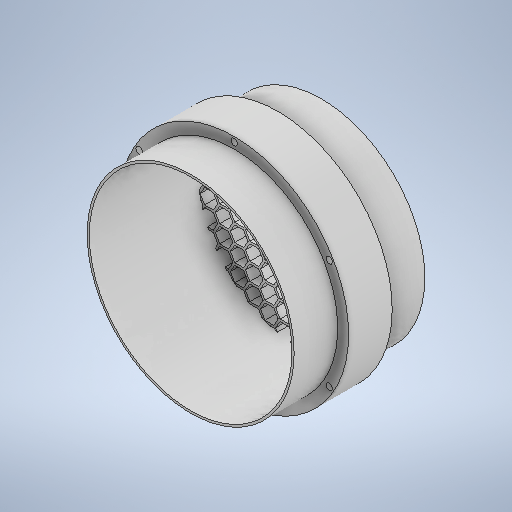
# Autodesk Inventor part: felga
Saved by Autodesk Inventor 2025.3 (Build 293356000, 356)
## iProperties
Created: 2026-03-06
Part Number: felga
Material: Generic
Document SubType Name: Modeling
Designer: ksawe
Density: 1 g/cm^3
Appearance: Default
Author: ksawe
Autodesk Inventor part; units mm, degrees
(part 1 of 2)
ref_plane "YZ Plane" through (0, 0, 0) normal (1, 0, 0) x (0, 1, 0)
ref_plane "XZ Plane" through (0, 0, 0) normal (0, 1, 0) x (-1, 0, 0)
sketch "Sketch8" plane through (0, 0, 0) normal (0, 0, 1) x (1, 0, 0)
  circle A0 centre (0, 0) radius 47.5
  dimension "d29" = 95
  constraints: 1 centre point, 1 coincident
  measures "d29" diameter of A0
extrude "Extrusion5" add sketch "Sketch8" along normal blind 60
ref_plane "Work Plane2" through (0, 0, 30) normal (0, 0, 1) x (1, 0, 0)
sketch "Sketch9" plane through (0, 0, 30) normal (0, 0, 1) x (1, 0, 0)
  circle A0 centre (0, 0) radius 52.5
  dimension "d33" = 105
  constraints: 1 centre point, 1 coincident
  measures "d33" diameter of A0
extrude "Extrusion6" add sketch "Sketch9" along normal mid plane 20
sketch "Sketch10" plane through (0, 0, 60) normal (0, 0, 1) x (1, 0, 0)
  circle A0 centre (0, 0) radius 46.5
  dimension "d36" = 93
  constraints: 1 centre point, 1 coincident
  measures "d36" diameter of A0
extrude "Extrusion7" cut sketch "Sketch10" against normal blind 50
sketch "Sketch14" plane through (0, 0, 0) normal (0, 0, -1) x (-1, 0, 0)
  line L0 (-2.0283, -3.4956) -> (-4.0414, 0.0088)
  line L1 (-4.0414, 0.0088) -> (-2.0131, 3.5044)
  line L2 (-2.0131, 3.5044) -> (2.0283, 3.4956)
  line L3 (2.0283, 3.4956) -> (4.0414, -0.0088)
  line L4 (4.0414, -0.0088) -> (2.0131, -3.5044)
  line L5 (2.0131, -3.5044) -> (-2.0283, -3.4956)
  line L6 (0, 0) -> (8.9984, 0) construction
  line L7 (0, 3.5) -> (0, 12.1066)
  line L8 (3.0311, -1.75) -> (7.7928, -4.4992)
  line L9 (4.0414, 7.9912) -> (2.0131, 4.4956)
  line L10 (2.0283, 11.4956) -> (4.0414, 7.9912)
  line L11 (-2.0131, 11.5044) -> (2.0283, 11.4956)
  line L12 (-4.0414, 8.0088) -> (-2.0131, 11.5044)
  line L13 (-2.0283, 4.5044) -> (-4.0414, 8.0088)
  line L14 (2.0131, 4.4956) -> (-2.0283, 4.5044)
  line L15 (4.0414, -8.0088) -> (2.0131, -11.5044)
  line L16 (2.0283, -4.5044) -> (4.0414, -8.0088)
  line L17 (-2.0131, -4.4956) -> (2.0283, -4.5044)
  line L18 (-4.0414, -7.9912) -> (-2.0131, -4.4956)
  line L19 (-2.0283, -11.4956) -> (-4.0414, -7.9912)
  line L20 (2.0131, -11.5044) -> (-2.0283, -11.4956)
  line L21 (4.0414, 15.9912) -> (2.0131, 12.4956)
  line L22 (2.0283, 19.4956) -> (4.0414, 15.9912)
  line L23 (-2.0131, 19.5044) -> (2.0283, 19.4956)
  line L24 (-4.0414, 16.0088) -> (-2.0131, 19.5044)
  line L25 (-2.0283, 12.5044) -> (-4.0414, 16.0088)
  line L26 (2.0131, 12.4956) -> (-2.0283, 12.5044)
  line L27 (4.0414, -16.0088) -> (2.0131, -19.5044)
  line L28 (2.0283, -12.5044) -> (4.0414, -16.0088)
  line L29 (-2.0131, -12.4956) -> (2.0283, -12.5044)
  line L30 (-4.0414, -15.9912) -> (-2.0131, -12.4956)
  line L31 (-2.0283, -19.4956) -> (-4.0414, -15.9912)
  line L32 (2.0131, -19.5044) -> (-2.0283, -19.4956)
  line L33 (4.0414, 23.9912) -> (2.0131, 20.4956)
  line L34 (2.0283, 27.4956) -> (4.0414, 23.9912)
  line L35 (-2.0131, 27.5044) -> (2.0283, 27.4956)
  line L36 (-4.0414, 24.0088) -> (-2.0131, 27.5044)
  line L37 (-2.0283, 20.5044) -> (-4.0414, 24.0088)
  line L38 (2.0131, 20.4956) -> (-2.0283, 20.5044)
  line L39 (4.0414, -24.0088) -> (2.0131, -27.5044)
  line L40 (2.0283, -20.5044) -> (4.0414, -24.0088)
  line L41 (-2.0131, -20.4956) -> (2.0283, -20.5044)
  line L42 (-4.0414, -23.9912) -> (-2.0131, -20.4956)
  line L43 (-2.0283, -27.4956) -> (-4.0414, -23.9912)
  line L44 (2.0131, -27.5044) -> (-2.0283, -27.4956)
  line L45 (4.0414, 31.9912) -> (2.0131, 28.4956)
  line L46 (2.0283, 35.4956) -> (4.0414, 31.9912)
  line L47 (-2.0131, 35.5044) -> (2.0283, 35.4956)
  line L48 (-4.0414, 32.0088) -> (-2.0131, 35.5044)
  line L49 (-2.0283, 28.5044) -> (-4.0414, 32.0088)
  line L50 (2.0131, 28.4956) -> (-2.0283, 28.5044)
  line L51 (4.0414, -32.0088) -> (2.0131, -35.5044)
  line L52 (2.0283, -28.5044) -> (4.0414, -32.0088)
  line L53 (-2.0131, -28.4956) -> (2.0283, -28.5044)
  line L54 (-4.0414, -31.9912) -> (-2.0131, -28.4956)
  line L55 (-2.0283, -35.4956) -> (-4.0414, -31.9912)
  line L56 (2.0131, -35.5044) -> (-2.0283, -35.4956)
  line L57 (4.0414, 39.9912) -> (2.0131, 36.4956)
  line L58 (2.0283, 43.4956) -> (4.0414, 39.9912)
  line L59 (-2.0131, 43.5044) -> (2.0283, 43.4956)
  line L60 (-4.0414, 40.0088) -> (-2.0131, 43.5044)
  line L61 (-2.0283, 36.5044) -> (-4.0414, 40.0088)
  line L62 (2.0131, 36.4956) -> (-2.0283, 36.5044)
  line L63 (4.0414, -40.0088) -> (2.0131, -43.5044)
  line L64 (2.0283, -36.5044) -> (4.0414, -40.0088)
  line L65 (-2.0131, -36.4956) -> (2.0283, -36.5044)
  line L66 (-4.0414, -39.9912) -> (-2.0131, -36.4956)
  line L67 (-2.0283, -43.4956) -> (-4.0414, -39.9912)
  line L68 (2.0131, -43.5044) -> (-2.0283, -43.4956)
  line L69 (4.0414, 47.9912) -> (2.0131, 44.4956)
  line L70 (2.0283, 51.4956) -> (4.0414, 47.9912)
  line L71 (-2.0131, 51.5044) -> (2.0283, 51.4956)
  line L72 (-4.0414, 48.0088) -> (-2.0131, 51.5044)
  line L73 (-2.0283, 44.5044) -> (-4.0414, 48.0088)
  line L74 (2.0131, 44.4956) -> (-2.0283, 44.5044)
  line L75 (4.0414, -48.0088) -> (2.0131, -51.5044)
  line L76 (2.0283, -44.5044) -> (4.0414, -48.0088)
  line L77 (-2.0131, -44.4956) -> (2.0283, -44.5044)
  line L78 (-4.0414, -47.9912) -> (-2.0131, -44.4956)
  line L79 (-2.0283, -51.4956) -> (-4.0414, -47.9912)
  line L80 (2.0131, -51.5044) -> (-2.0283, -51.4956)
  line L81 (4.0414, 55.9912) -> (2.0131, 52.4956)
  line L82 (2.0283, 59.4956) -> (4.0414, 55.9912)
  line L83 (-2.0131, 59.5044) -> (2.0283, 59.4956)
  line L84 (-4.0414, 56.0088) -> (-2.0131, 59.5044)
  line L85 (-2.0283, 52.5044) -> (-4.0414, 56.0088)
  line L86 (2.0131, 52.4956) -> (-2.0283, 52.5044)
  line L87 (4.0414, -56.0088) -> (2.0131, -59.5044)
  line L88 (2.0283, -52.5044) -> (4.0414, -56.0088)
  line L89 (-2.0131, -52.4956) -> (2.0283, -52.5044)
  line L90 (-4.0414, -55.9912) -> (-2.0131, -52.4956)
  line L91 (-2.0283, -59.4956) -> (-4.0414, -55.9912)
  line L92 (2.0131, -59.5044) -> (-2.0283, -59.4956)
  line L93 (10.9696, -4.0088) -> (8.9413, -7.5044)
  line L94 (8.9565, -0.5044) -> (10.9696, -4.0088)
  line L95 (4.9151, -0.4956) -> (8.9565, -0.5044)
  line L96 (2.8868, -3.9912) -> (4.9151, -0.4956)
  line L97 (4.8999, -7.4956) -> (2.8868, -3.9912)
  line L98 (8.9413, -7.5044) -> (4.8999, -7.4956)
  line L99 (10.9696, 3.9912) -> (8.9413, 0.4956)
  line L100 (8.9565, 7.4956) -> (10.9696, 3.9912)
  line L101 (4.9151, 7.5044) -> (8.9565, 7.4956)
  line L102 (2.8868, 4.0088) -> (4.9151, 7.5044)
  line L103 (4.8999, 0.5044) -> (2.8868, 4.0088)
  line L104 (8.9413, 0.4956) -> (4.8999, 0.5044)
  line L105 (10.9696, -12.0088) -> (8.9413, -15.5044)
  line L106 (8.9565, -8.5044) -> (10.9696, -12.0088)
  line L107 (4.9151, -8.4956) -> (8.9565, -8.5044)
  line L108 (2.8868, -11.9912) -> (4.9151, -8.4956)
  line L109 (4.8999, -15.4956) -> (2.8868, -11.9912)
  line L110 (8.9413, -15.5044) -> (4.8999, -15.4956)
  line L111 (10.9696, 11.9912) -> (8.9413, 8.4956)
  line L112 (8.9565, 15.4956) -> (10.9696, 11.9912)
  line L113 (4.9151, 15.5044) -> (8.9565, 15.4956)
  line L114 (2.8868, 12.0088) -> (4.9151, 15.5044)
  line L115 (4.8999, 8.5044) -> (2.8868, 12.0088)
  line L116 (8.9413, 8.4956) -> (4.8999, 8.5044)
  line L117 (10.9696, -20.0088) -> (8.9413, -23.5044)
  line L118 (8.9565, -16.5044) -> (10.9696, -20.0088)
  line L119 (4.9151, -16.4956) -> (8.9565, -16.5044)
  line L120 (2.8868, -19.9912) -> (4.9151, -16.4956)
  line L121 (4.8999, -23.4956) -> (2.8868, -19.9912)
  line L122 (8.9413, -23.5044) -> (4.8999, -23.4956)
  line L123 (10.9696, 19.9912) -> (8.9413, 16.4956)
  line L124 (8.9565, 23.4956) -> (10.9696, 19.9912)
  line L125 (4.9151, 23.5044) -> (8.9565, 23.4956)
  line L126 (2.8868, 20.0088) -> (4.9151, 23.5044)
  line L127 (4.8999, 16.5044) -> (2.8868, 20.0088)
  line L128 (8.9413, 16.4956) -> (4.8999, 16.5044)
  line L129 (10.9696, -28.0088) -> (8.9413, -31.5044)
  line L130 (8.9565, -24.5044) -> (10.9696, -28.0088)
  line L131 (4.9151, -24.4956) -> (8.9565, -24.5044)
  line L132 (2.8868, -27.9912) -> (4.9151, -24.4956)
  line L133 (4.8999, -31.4956) -> (2.8868, -27.9912)
  line L134 (8.9413, -31.5044) -> (4.8999, -31.4956)
  line L135 (10.9696, 27.9912) -> (8.9413, 24.4956)
  line L136 (8.9565, 31.4956) -> (10.9696, 27.9912)
  line L137 (4.9151, 31.5044) -> (8.9565, 31.4956)
  line L138 (2.8868, 28.0088) -> (4.9151, 31.5044)
  line L139 (4.8999, 24.5044) -> (2.8868, 28.0088)
  line L140 (8.9413, 24.4956) -> (4.8999, 24.5044)
  line L141 (10.9696, -36.0088) -> (8.9413, -39.5044)
  line L142 (8.9565, -32.5044) -> (10.9696, -36.0088)
  line L143 (4.9151, -32.4956) -> (8.9565, -32.5044)
  line L144 (2.8868, -35.9912) -> (4.9151, -32.4956)
  line L145 (4.8999, -39.4956) -> (2.8868, -35.9912)
  line L146 (8.9413, -39.5044) -> (4.8999, -39.4956)
  line L147 (10.9696, 35.9912) -> (8.9413, 32.4956)
  line L148 (8.9565, 39.4956) -> (10.9696, 35.9912)
  line L149 (4.9151, 39.5044) -> (8.9565, 39.4956)
  line L150 (2.8868, 36.0088) -> (4.9151, 39.5044)
  line L151 (4.8999, 32.5044) -> (2.8868, 36.0088)
  line L152 (8.9413, 32.4956) -> (4.8999, 32.5044)
  line L153 (10.9696, -44.0088) -> (8.9413, -47.5044)
  line L154 (8.9565, -40.5044) -> (10.9696, -44.0088)
  line L155 (4.9151, -40.4956) -> (8.9565, -40.5044)
  line L156 (2.8868, -43.9912) -> (4.9151, -40.4956)
  line L157 (4.8999, -47.4956) -> (2.8868, -43.9912)
  line L158 (8.9413, -47.5044) -> (4.8999, -47.4956)
  line L159 (10.9696, 43.9912) -> (8.9413, 40.4956)
  line L160 (8.9565, 47.4956) -> (10.9696, 43.9912)
  line L161 (4.9151, 47.5044) -> (8.9565, 47.4956)
  line L162 (2.8868, 44.0088) -> (4.9151, 47.5044)
  line L163 (4.8999, 40.5044) -> (2.8868, 44.0088)
  line L164 (8.9413, 40.4956) -> (4.8999, 40.5044)
  line L165 (10.9696, -52.0088) -> (8.9413, -55.5044)
  line L166 (8.9565, -48.5044) -> (10.9696, -52.0088)
  line L167 (4.9151, -48.4956) -> (8.9565, -48.5044)
  line L168 (2.8868, -51.9912) -> (4.9151, -48.4956)
  line L169 (4.8999, -55.4956) -> (2.8868, -51.9912) construction
  line L170 (8.9413, -55.5044) -> (4.8999, -55.4956)
  line L171 (10.9696, 51.9912) -> (8.9413, 48.4956)
  line L172 (8.9565, 55.4956) -> (10.9696, 51.9912)
  line L173 (4.9151, 55.5044) -> (8.9565, 55.4956)
  line L174 (2.8868, 52.0088) -> (4.9151, 55.5044)
  line L175 (4.8999, 48.5044) -> (2.8868, 52.0088)
  line L176 (8.9413, 48.4956) -> (4.8999, 48.5044)
  line L177 (10.9696, -60.0088) -> (8.9413, -63.5044)
  line L178 (8.9565, -56.5044) -> (10.9696, -60.0088)
  line L179 (4.9151, -56.4956) -> (8.9565, -56.5044)
  line L180 (2.8868, -59.9912) -> (4.9151, -56.4956)
  line L181 (4.8999, -63.4956) -> (2.8868, -59.9912)
  line L182 (8.9413, -63.5044) -> (4.8999, -63.4956)
  line L183 (-2.8868, 3.9912) -> (-4.9151, 0.4956)
  line L184 (-4.8999, 7.4956) -> (-2.8868, 3.9912)
  line L185 (-8.9413, 7.5044) -> (-4.8999, 7.4956)
  line L186 (-10.9696, 4.0088) -> (-8.9413, 7.5044)
  line L187 (-8.9565, 0.5044) -> (-10.9696, 4.0088)
  line L188 (-4.9151, 0.4956) -> (-8.9565, 0.5044)
  line L189 (-2.8868, 11.9912) -> (-4.9151, 8.4956)
  line L190 (-4.8999, 15.4956) -> (-2.8868, 11.9912)
  line L191 (-8.9413, 15.5044) -> (-4.8999, 15.4956)
  line L192 (-10.9696, 12.0088) -> (-8.9413, 15.5044)
  line L193 (-8.9565, 8.5044) -> (-10.9696, 12.0088)
  line L194 (-4.9151, 8.4956) -> (-8.9565, 8.5044)
  line L195 (-2.8868, -4.0088) -> (-4.9151, -7.5044)
  line L196 (-4.8999, -0.5044) -> (-2.8868, -4.0088)
  line L197 (-8.9413, -0.4956) -> (-4.8999, -0.5044)
  line L198 (-10.9696, -3.9912) -> (-8.9413, -0.4956)
  line L199 (-8.9565, -7.4956) -> (-10.9696, -3.9912)
  line L200 (-4.9151, -7.5044) -> (-8.9565, -7.4956)
  line L201 (-2.8868, 19.9912) -> (-4.9151, 16.4956)
  line L202 (-4.8999, 23.4956) -> (-2.8868, 19.9912)
  line L203 (-8.9413, 23.5044) -> (-4.8999, 23.4956)
  line L204 (-10.9696, 20.0088) -> (-8.9413, 23.5044)
  line L205 (-8.9565, 16.5044) -> (-10.9696, 20.0088)
  line L206 (-4.9151, 16.4956) -> (-8.9565, 16.5044)
  line L207 (-2.8868, -12.0088) -> (-4.9151, -15.5044)
  line L208 (-4.8999, -8.5044) -> (-2.8868, -12.0088)
  line L209 (-8.9413, -8.4956) -> (-4.8999, -8.5044)
  line L210 (-10.9696, -11.9912) -> (-8.9413, -8.4956)
  line L211 (-8.9565, -15.4956) -> (-10.9696, -11.9912)
  line L212 (-4.9151, -15.5044) -> (-8.9565, -15.4956)
  line L213 (-2.8868, 27.9912) -> (-4.9151, 24.4956)
  line L214 (-4.8999, 31.4956) -> (-2.8868, 27.9912)
  line L215 (-8.9413, 31.5044) -> (-4.8999, 31.4956)
  line L216 (-10.9696, 28.0088) -> (-8.9413, 31.5044)
  line L217 (-8.9565, 24.5044) -> (-10.9696, 28.0088)
  line L218 (-4.9151, 24.4956) -> (-8.9565, 24.5044)
  line L219 (-2.8868, -20.0088) -> (-4.9151, -23.5044)
  line L220 (-4.8999, -16.5044) -> (-2.8868, -20.0088)
  line L221 (-8.9413, -16.4956) -> (-4.8999, -16.5044)
  line L222 (-10.9696, -19.9912) -> (-8.9413, -16.4956)
  line L223 (-8.9565, -23.4956) -> (-10.9696, -19.9912)
  line L224 (-4.9151, -23.5044) -> (-8.9565, -23.4956)
  line L225 (-2.8868, 35.9912) -> (-4.9151, 32.4956)
  line L226 (-4.8999, 39.4956) -> (-2.8868, 35.9912)
  line L227 (-8.9413, 39.5044) -> (-4.8999, 39.4956)
  line L228 (-10.9696, 36.0088) -> (-8.9413, 39.5044)
  line L229 (-8.9565, 32.5044) -> (-10.9696, 36.0088)
  line L230 (-4.9151, 32.4956) -> (-8.9565, 32.5044)
  line L231 (-2.8868, -28.0088) -> (-4.9151, -31.5044)
  line L232 (-4.8999, -24.5044) -> (-2.8868, -28.0088)
  line L233 (-8.9413, -24.4956) -> (-4.8999, -24.5044)
  line L234 (-10.9696, -27.9912) -> (-8.9413, -24.4956)
  line L235 (-8.9565, -31.4956) -> (-10.9696, -27.9912)
  line L236 (-4.9151, -31.5044) -> (-8.9565, -31.4956)
  line L237 (-2.8868, 43.9912) -> (-4.9151, 40.4956)
  line L238 (-4.8999, 47.4956) -> (-2.8868, 43.9912)
  line L239 (-8.9413, 47.5044) -> (-4.8999, 47.4956)
  line L240 (-10.9696, 44.0088) -> (-8.9413, 47.5044)
  line L241 (-8.9565, 40.5044) -> (-10.9696, 44.0088)
  line L242 (-4.9151, 40.4956) -> (-8.9565, 40.5044)
  line L243 (-2.8868, -36.0088) -> (-4.9151, -39.5044)
  line L244 (-4.8999, -32.5044) -> (-2.8868, -36.0088)
  line L245 (-8.9413, -32.4956) -> (-4.8999, -32.5044)
  line L246 (-10.9696, -35.9912) -> (-8.9413, -32.4956)
  line L247 (-8.9565, -39.4956) -> (-10.9696, -35.9912)
  line L248 (-4.9151, -39.5044) -> (-8.9565, -39.4956)
  line L249 (-2.8868, 51.9912) -> (-4.9151, 48.4956)
  line L250 (-4.8999, 55.4956) -> (-2.8868, 51.9912)
  line L251 (-8.9413, 55.5044) -> (-4.8999, 55.4956)
  line L252 (-10.9696, 52.0088) -> (-8.9413, 55.5044)
  line L253 (-8.9565, 48.5044) -> (-10.9696, 52.0088)
  line L254 (-4.9151, 48.4956) -> (-8.9565, 48.5044)
  line L255 (-2.8868, -44.0088) -> (-4.9151, -47.5044)
  line L256 (-4.8999, -40.5044) -> (-2.8868, -44.0088)
  line L257 (-8.9413, -40.4956) -> (-4.8999, -40.5044)
  line L258 (-10.9696, -43.9912) -> (-8.9413, -40.4956)
  line L259 (-8.9565, -47.4956) -> (-10.9696, -43.9912)
  line L260 (-4.9151, -47.5044) -> (-8.9565, -47.4956)
  line L261 (-2.8868, 59.9912) -> (-4.9151, 56.4956)
  line L262 (-4.8999, 63.4956) -> (-2.8868, 59.9912)
  line L263 (-8.9413, 63.5044) -> (-4.8999, 63.4956)
  line L264 (-10.9696, 60.0088) -> (-8.9413, 63.5044)
  line L265 (-8.9565, 56.5044) -> (-10.9696, 60.0088)
  line L266 (-4.9151, 56.4956) -> (-8.9565, 56.5044)
  line L267 (-2.8868, -52.0088) -> (-4.9151, -55.5044)
  line L268 (-4.8999, -48.5044) -> (-2.8868, -52.0088)
  line L269 (-8.9413, -48.4956) -> (-4.8999, -48.5044)
  line L270 (-10.9696, -51.9912) -> (-8.9413, -48.4956)
  line L271 (-8.9565, -55.4956) -> (-10.9696, -51.9912)
  line L272 (-4.9151, -55.5044) -> (-8.9565, -55.4956)
  line L273 (17.8978, -8.0088) -> (15.8695, -11.5044)
  line L274 (15.8847, -4.5044) -> (17.8978, -8.0088)
  line L275 (11.8433, -4.4956) -> (15.8847, -4.5044)
  line L276 (9.815, -7.9912) -> (11.8433, -4.4956)
  line L277 (11.8281, -11.4956) -> (9.815, -7.9912)
  line L278 (15.8695, -11.5044) -> (11.8281, -11.4956)
  line L279 (17.8978, -0.0088) -> (15.8695, -3.5044)
  line L280 (15.8847, 3.4956) -> (17.8978, -0.0088)
  line L281 (11.8433, 3.5044) -> (15.8847, 3.4956)
  line L282 (9.815, 0.0088) -> (11.8433, 3.5044)
  line L283 (11.8281, -3.4956) -> (9.815, 0.0088)
  line L284 (15.8695, -3.5044) -> (11.8281, -3.4956)
  line L285 (17.8978, -16.0088) -> (15.8695, -19.5044)
  line L286 (15.8847, -12.5044) -> (17.8978, -16.0088)
  line L287 (11.8433, -12.4956) -> (15.8847, -12.5044)
  line L288 (9.815, -15.9912) -> (11.8433, -12.4956)
  line L289 (11.8281, -19.4956) -> (9.815, -15.9912)
  line L290 (15.8695, -19.5044) -> (11.8281, -19.4956)
  line L291 (17.8978, 7.9912) -> (15.8695, 4.4956)
  line L292 (15.8847, 11.4956) -> (17.8978, 7.9912)
  line L293 (11.8433, 11.5044) -> (15.8847, 11.4956)
  line L294 (9.815, 8.0088) -> (11.8433, 11.5044)
  line L295 (11.8281, 4.5044) -> (9.815, 8.0088)
  line L296 (15.8695, 4.4956) -> (11.8281, 4.5044)
  line L297 (17.8978, -24.0088) -> (15.8695, -27.5044)
  line L298 (15.8847, -20.5044) -> (17.8978, -24.0088)
  line L299 (11.8433, -20.4956) -> (15.8847, -20.5044)
  line L300 (9.815, -23.9912) -> (11.8433, -20.4956)
  line L301 (11.8281, -27.4956) -> (9.815, -23.9912)
  line L302 (15.8695, -27.5044) -> (11.8281, -27.4956)
  line L303 (17.8978, 15.9912) -> (15.8695, 12.4956)
  line L304 (15.8847, 19.4956) -> (17.8978, 15.9912)
  line L305 (11.8433, 19.5044) -> (15.8847, 19.4956)
  line L306 (9.815, 16.0088) -> (11.8433, 19.5044)
  line L307 (11.8281, 12.5044) -> (9.815, 16.0088)
  line L308 (15.8695, 12.4956) -> (11.8281, 12.5044)
  line L309 (17.8978, -32.0088) -> (15.8695, -35.5044)
  line L310 (15.8847, -28.5044) -> (17.8978, -32.0088)
  line L311 (11.8433, -28.4956) -> (15.8847, -28.5044)
  line L312 (9.815, -31.9912) -> (11.8433, -28.4956)
  line L313 (11.8281, -35.4956) -> (9.815, -31.9912)
  line L314 (15.8695, -35.5044) -> (11.8281, -35.4956)
  line L315 (17.8978, 23.9912) -> (15.8695, 20.4956)
  line L316 (15.8847, 27.4956) -> (17.8978, 23.9912)
  line L317 (11.8433, 27.5044) -> (15.8847, 27.4956)
  line L318 (9.815, 24.0088) -> (11.8433, 27.5044)
  line L319 (11.8281, 20.5044) -> (9.815, 24.0088)
  line L320 (15.8695, 20.4956) -> (11.8281, 20.5044)
  line L321 (17.8978, -40.0088) -> (15.8695, -43.5044)
  line L322 (15.8847, -36.5044) -> (17.8978, -40.0088)
  line L323 (11.8433, -36.4956) -> (15.8847, -36.5044)
  line L324 (9.815, -39.9912) -> (11.8433, -36.4956)
  line L325 (11.8281, -43.4956) -> (9.815, -39.9912)
  line L326 (15.8695, -43.5044) -> (11.8281, -43.4956)
  line L327 (17.8978, 31.9912) -> (15.8695, 28.4956)
  line L328 (15.8847, 35.4956) -> (17.8978, 31.9912)
  line L329 (11.8433, 35.5044) -> (15.8847, 35.4956)
  line L330 (9.815, 32.0088) -> (11.8433, 35.5044)
  line L331 (11.8281, 28.5044) -> (9.815, 32.0088)
  line L332 (15.8695, 28.4956) -> (11.8281, 28.5044)
  line L333 (17.8978, -48.0088) -> (15.8695, -51.5044)
  line L334 (15.8847, -44.5044) -> (17.8978, -48.0088)
  line L335 (11.8433, -44.4956) -> (15.8847, -44.5044)
  line L336 (9.815, -47.9912) -> (11.8433, -44.4956)
  line L337 (11.8281, -51.4956) -> (9.815, -47.9912)
  line L338 (15.8695, -51.5044) -> (11.8281, -51.4956)
  line L339 (17.8978, 39.9912) -> (15.8695, 36.4956)
  line L340 (15.8847, 43.4956) -> (17.8978, 39.9912)
  line L341 (11.8433, 43.5044) -> (15.8847, 43.4956)
  line L342 (9.815, 40.0088) -> (11.8433, 43.5044)
  line L343 (11.8281, 36.5044) -> (9.815, 40.0088)
  line L344 (15.8695, 36.4956) -> (11.8281, 36.5044)
  line L345 (17.8978, -56.0088) -> (15.8695, -59.5044)
  line L346 (15.8847, -52.5044) -> (17.8978, -56.0088)
  line L347 (11.8433, -52.4956) -> (15.8847, -52.5044)
  line L348 (9.815, -55.9912) -> (11.8433, -52.4956)
  line L349 (11.8281, -59.4956) -> (9.815, -55.9912)
  line L350 (15.8695, -59.5044) -> (11.8281, -59.4956)
  line L351 (17.8978, 47.9912) -> (15.8695, 44.4956)
  line L352 (15.8847, 51.4956) -> (17.8978, 47.9912)
  line L353 (11.8433, 51.5044) -> (15.8847, 51.4956)
  line L354 (9.815, 48.0088) -> (11.8433, 51.5044)
  line L355 (11.8281, 44.5044) -> (9.815, 48.0088)
  line L356 (15.8695, 44.4956) -> (11.8281, 44.5044)
  line L357 (17.8978, -64.0088) -> (15.8695, -67.5044)
  line L358 (15.8847, -60.5044) -> (17.8978, -64.0088)
  line L359 (11.8433, -60.4956) -> (15.8847, -60.5044)
  line L360 (9.815, -63.9912) -> (11.8433, -60.4956)
  line L361 (11.8281, -67.4956) -> (9.815, -63.9912)
  line L362 (15.8695, -67.5044) -> (11.8281, -67.4956)
  line L363 (-9.815, 7.9912) -> (-11.8433, 4.4956)
  line L364 (-11.8281, 11.4956) -> (-9.815, 7.9912)
  line L365 (-15.8695, 11.5044) -> (-11.8281, 11.4956)
  line L366 (-17.8978, 8.0088) -> (-15.8695, 11.5044)
  line L367 (-15.8847, 4.5044) -> (-17.8978, 8.0088)
  line L368 (-11.8433, 4.4956) -> (-15.8847, 4.5044)
  line L369 (-9.815, 15.9912) -> (-11.8433, 12.4956)
  line L370 (-11.8281, 19.4956) -> (-9.815, 15.9912)
  line L371 (-15.8695, 19.5044) -> (-11.8281, 19.4956)
  line L372 (-17.8978, 16.0088) -> (-15.8695, 19.5044)
  line L373 (-15.8847, 12.5044) -> (-17.8978, 16.0088)
  line L374 (-11.8433, 12.4956) -> (-15.8847, 12.5044)
  line L375 (-9.815, -0.0088) -> (-11.8433, -3.5044)
  line L376 (-11.8281, 3.4956) -> (-9.815, -0.0088)
  line L377 (-15.8695, 3.5044) -> (-11.8281, 3.4956)
  line L378 (-17.8978, 0.0088) -> (-15.8695, 3.5044)
  line L379 (-15.8847, -3.4956) -> (-17.8978, 0.0088)
  line L380 (-11.8433, -3.5044) -> (-15.8847, -3.4956)
  line L381 (-9.815, 23.9912) -> (-11.8433, 20.4956)
  line L382 (-11.8281, 27.4956) -> (-9.815, 23.9912)
  line L383 (-15.8695, 27.5044) -> (-11.8281, 27.4956)
  line L384 (-17.8978, 24.0088) -> (-15.8695, 27.5044)
  line L385 (-15.8847, 20.5044) -> (-17.8978, 24.0088)
  line L386 (-11.8433, 20.4956) -> (-15.8847, 20.5044)
  line L387 (-9.815, -8.0088) -> (-11.8433, -11.5044)
  line L388 (-11.8281, -4.5044) -> (-9.815, -8.0088)
  line L389 (-15.8695, -4.4956) -> (-11.8281, -4.5044)
  line L390 (-17.8978, -7.9912) -> (-15.8695, -4.4956)
  line L391 (-15.8847, -11.4956) -> (-17.8978, -7.9912)
  line L392 (-11.8433, -11.5044) -> (-15.8847, -11.4956)
  line L393 (-9.815, 31.9912) -> (-11.8433, 28.4956)
  line L394 (-11.8281, 35.4956) -> (-9.815, 31.9912)
  line L395 (-15.8695, 35.5044) -> (-11.8281, 35.4956)
  line L396 (-17.8978, 32.0088) -> (-15.8695, 35.5044)
  line L397 (-15.8847, 28.5044) -> (-17.8978, 32.0088)
  line L398 (-11.8433, 28.4956) -> (-15.8847, 28.5044)
  line L399 (-9.815, -16.0088) -> (-11.8433, -19.5044)
  line L400 (-11.8281, -12.5044) -> (-9.815, -16.0088)
  line L401 (-15.8695, -12.4956) -> (-11.8281, -12.5044)
  line L402 (-17.8978, -15.9912) -> (-15.8695, -12.4956)
  line L403 (-15.8847, -19.4956) -> (-17.8978, -15.9912)
  line L404 (-11.8433, -19.5044) -> (-15.8847, -19.4956)
  line L405 (-9.815, 39.9912) -> (-11.8433, 36.4956)
  line L406 (-11.8281, 43.4956) -> (-9.815, 39.9912)
  line L407 (-15.8695, 43.5044) -> (-11.8281, 43.4956)
  line L408 (-17.8978, 40.0088) -> (-15.8695, 43.5044)
  line L409 (-15.8847, 36.5044) -> (-17.8978, 40.0088)
  line L410 (-11.8433, 36.4956) -> (-15.8847, 36.5044)
  line L411 (-9.815, -24.0088) -> (-11.8433, -27.5044)
  line L412 (-11.8281, -20.5044) -> (-9.815, -24.0088)
  line L413 (-15.8695, -20.4956) -> (-11.8281, -20.5044)
  line L414 (-17.8978, -23.9912) -> (-15.8695, -20.4956)
  line L415 (-15.8847, -27.4956) -> (-17.8978, -23.9912)
  line L416 (-11.8433, -27.5044) -> (-15.8847, -27.4956)
  line L417 (-9.815, 47.9912) -> (-11.8433, 44.4956)
  line L418 (-11.8281, 51.4956) -> (-9.815, 47.9912)
  line L419 (-15.8695, 51.5044) -> (-11.8281, 51.4956)
  line L420 (-17.8978, 48.0088) -> (-15.8695, 51.5044)
  line L421 (-15.8847, 44.5044) -> (-17.8978, 48.0088)
  line L422 (-11.8433, 44.4956) -> (-15.8847, 44.5044)
  line L423 (-9.815, -32.0088) -> (-11.8433, -35.5044)
  line L424 (-11.8281, -28.5044) -> (-9.815, -32.0088)
  line L425 (-15.8695, -28.4956) -> (-11.8281, -28.5044)
  line L426 (-17.8978, -31.9912) -> (-15.8695, -28.4956)
  line L427 (-15.8847, -35.4956) -> (-17.8978, -31.9912)
  line L428 (-11.8433, -35.5044) -> (-15.8847, -35.4956)
  line L429 (-9.815, 55.9912) -> (-11.8433, 52.4956)
  line L430 (-11.8281, 59.4956) -> (-9.815, 55.9912)
  line L431 (-15.8695, 59.5044) -> (-11.8281, 59.4956)
  line L432 (-17.8978, 56.0088) -> (-15.8695, 59.5044)
  line L433 (-15.8847, 52.5044) -> (-17.8978, 56.0088)
  line L434 (-11.8433, 52.4956) -> (-15.8847, 52.5044)
  line L435 (-9.815, -40.0088) -> (-11.8433, -43.5044)
  line L436 (-11.8281, -36.5044) -> (-9.815, -40.0088)
  line L437 (-15.8695, -36.4956) -> (-11.8281, -36.5044)
  line L438 (-17.8978, -39.9912) -> (-15.8695, -36.4956)
  line L439 (-15.8847, -43.4956) -> (-17.8978, -39.9912)
  line L440 (-11.8433, -43.5044) -> (-15.8847, -43.4956)
  line L441 (-9.815, 63.9912) -> (-11.8433, 60.4956)
  line L442 (-11.8281, 67.4956) -> (-9.815, 63.9912)
  line L443 (-15.8695, 67.5044) -> (-11.8281, 67.4956)
  line L444 (-17.8978, 64.0088) -> (-15.8695, 67.5044)
  line L445 (-15.8847, 60.5044) -> (-17.8978, 64.0088)
  line L446 (-11.8433, 60.4956) -> (-15.8847, 60.5044)
  line L447 (-9.815, -48.0088) -> (-11.8433, -51.5044)
  line L448 (-11.8281, -44.5044) -> (-9.815, -48.0088)
  line L449 (-15.8695, -44.4956) -> (-11.8281, -44.5044)
  line L450 (-17.8978, -47.9912) -> (-15.8695, -44.4956)
  line L451 (-15.8847, -51.4956) -> (-17.8978, -47.9912)
  line L452 (-11.8433, -51.5044) -> (-15.8847, -51.4956)
  line L453 (24.8261, -12.0088) -> (22.7977, -15.5044)
  line L454 (22.8129, -8.5044) -> (24.8261, -12.0088)
  line L455 (18.7715, -8.4956) -> (22.8129, -8.5044)
  line L456 (16.7432, -11.9912) -> (18.7715, -8.4956)
  line L457 (18.7563, -15.4956) -> (16.7432, -11.9912)
  line L458 (22.7977, -15.5044) -> (18.7563, -15.4956)
  line L459 (24.8261, -4.0088) -> (22.7977, -7.5044)
  line L460 (22.8129, -0.5044) -> (24.8261, -4.0088)
  line L461 (18.7715, -0.4956) -> (22.8129, -0.5044)
  line L462 (16.7432, -3.9912) -> (18.7715, -0.4956)
  line L463 (18.7563, -7.4956) -> (16.7432, -3.9912)
  line L464 (22.7977, -7.5044) -> (18.7563, -7.4956)
  line L465 (24.8261, -20.0088) -> (22.7977, -23.5044)
  line L466 (22.8129, -16.5044) -> (24.8261, -20.0088)
  line L467 (18.7715, -16.4956) -> (22.8129, -16.5044)
  line L468 (16.7432, -19.9912) -> (18.7715, -16.4956)
  line L469 (18.7563, -23.4956) -> (16.7432, -19.9912)
  line L470 (22.7977, -23.5044) -> (18.7563, -23.4956)
  line L471 (24.8261, 3.9912) -> (22.7977, 0.4956)
  line L472 (22.8129, 7.4956) -> (24.8261, 3.9912)
  line L473 (18.7715, 7.5044) -> (22.8129, 7.4956)
  line L474 (16.7432, 4.0088) -> (18.7715, 7.5044)
  line L475 (18.7563, 0.5044) -> (16.7432, 4.0088)
  line L476 (22.7977, 0.4956) -> (18.7563, 0.5044)
  line L477 (24.8261, -28.0088) -> (22.7977, -31.5044)
  line L478 (22.8129, -24.5044) -> (24.8261, -28.0088)
  line L479 (18.7715, -24.4956) -> (22.8129, -24.5044)
  line L480 (16.7432, -27.9912) -> (18.7715, -24.4956)
  line L481 (18.7563, -31.4956) -> (16.7432, -27.9912)
  line L482 (22.7977, -31.5044) -> (18.7563, -31.4956)
  line L483 (24.8261, 11.9912) -> (22.7977, 8.4956)
  line L484 (22.8129, 15.4956) -> (24.8261, 11.9912)
  line L485 (18.7715, 15.5044) -> (22.8129, 15.4956)
  line L486 (16.7432, 12.0088) -> (18.7715, 15.5044)
  line L487 (18.7563, 8.5044) -> (16.7432, 12.0088)
  line L488 (22.7977, 8.4956) -> (18.7563, 8.5044)
  line L489 (24.8261, -36.0088) -> (22.7977, -39.5044)
  line L490 (22.8129, -32.5044) -> (24.8261, -36.0088)
  line L491 (18.7715, -32.4956) -> (22.8129, -32.5044)
  line L492 (16.7432, -35.9912) -> (18.7715, -32.4956)
  line L493 (18.7563, -39.4956) -> (16.7432, -35.9912)
  line L494 (22.7977, -39.5044) -> (18.7563, -39.4956)
  line L495 (24.8261, 19.9912) -> (22.7977, 16.4956)
  line L496 (22.8129, 23.4956) -> (24.8261, 19.9912)
  line L497 (18.7715, 23.5044) -> (22.8129, 23.4956)
  line L498 (16.7432, 20.0088) -> (18.7715, 23.5044)
  line L499 (18.7563, 16.5044) -> (16.7432, 20.0088)
  line L500 (22.7977, 16.4956) -> (18.7563, 16.5044)
  line L501 (24.8261, -44.0088) -> (22.7977, -47.5044)
  line L502 (22.8129, -40.5044) -> (24.8261, -44.0088)
  line L503 (18.7715, -40.4956) -> (22.8129, -40.5044)
  line L504 (16.7432, -43.9912) -> (18.7715, -40.4956)
  line L505 (18.7563, -47.4956) -> (16.7432, -43.9912)
  line L506 (22.7977, -47.5044) -> (18.7563, -47.4956)
  line L507 (24.8261, 27.9912) -> (22.7977, 24.4956)
  line L508 (22.8129, 31.4956) -> (24.8261, 27.9912)
  line L509 (18.7715, 31.5044) -> (22.8129, 31.4956)
  line L510 (16.7432, 28.0088) -> (18.7715, 31.5044)
  line L511 (18.7563, 24.5044) -> (16.7432, 28.0088)
  line L512 (22.7977, 24.4956) -> (18.7563, 24.5044)
  line L513 (24.8261, -52.0088) -> (22.7977, -55.5044)
  line L514 (22.8129, -48.5044) -> (24.8261, -52.0088)
  line L515 (18.7715, -48.4956) -> (22.8129, -48.5044)
  line L516 (16.7432, -51.9912) -> (18.7715, -48.4956)
  line L517 (18.7563, -55.4956) -> (16.7432, -51.9912)
  line L518 (22.7977, -55.5044) -> (18.7563, -55.4956)
  line L519 (24.8261, 35.9912) -> (22.7977, 32.4956)
  line L520 (22.8129, 39.4956) -> (24.8261, 35.9912)
  line L521 (18.7715, 39.5044) -> (22.8129, 39.4956)
  line L522 (16.7432, 36.0088) -> (18.7715, 39.5044)
  line L523 (18.7563, 32.5044) -> (16.7432, 36.0088)
  line L524 (22.7977, 32.4956) -> (18.7563, 32.5044)
  line L525 (24.8261, -60.0088) -> (22.7977, -63.5044)
  line L526 (22.8129, -56.5044) -> (24.8261, -60.0088)
  line L527 (18.7715, -56.4956) -> (22.8129, -56.5044)
  line L528 (16.7432, -59.9912) -> (18.7715, -56.4956)
  line L529 (18.7563, -63.4956) -> (16.7432, -59.9912)
  line L530 (22.7977, -63.5044) -> (18.7563, -63.4956)
  line L531 (24.8261, 43.9912) -> (22.7977, 40.4956)
  line L532 (22.8129, 47.4956) -> (24.8261, 43.9912)
  line L533 (18.7715, 47.5044) -> (22.8129, 47.4956)
  line L534 (16.7432, 44.0088) -> (18.7715, 47.5044)
  line L535 (18.7563, 40.5044) -> (16.7432, 44.0088)
  line L536 (22.7977, 40.4956) -> (18.7563, 40.5044)
  line L537 (24.8261, -68.0088) -> (22.7977, -71.5044)
  line L538 (22.8129, -64.5044) -> (24.8261, -68.0088)
  line L539 (18.7715, -64.4956) -> (22.8129, -64.5044)
  line L540 (16.7432, -67.9912) -> (18.7715, -64.4956)
  line L541 (18.7563, -71.4956) -> (16.7432, -67.9912)
  line L542 (22.7977, -71.5044) -> (18.7563, -71.4956)
  line L543 (-16.7432, 11.9912) -> (-18.7715, 8.4956)
  line L544 (-18.7563, 15.4956) -> (-16.7432, 11.9912)
  line L545 (-22.7977, 15.5044) -> (-18.7563, 15.4956)
  line L546 (-24.8261, 12.0088) -> (-22.7977, 15.5044)
  line L547 (-22.8129, 8.5044) -> (-24.8261, 12.0088)
  line L548 (-18.7715, 8.4956) -> (-22.8129, 8.5044)
  line L549 (-16.7432, 19.9912) -> (-18.7715, 16.4956)
  line L550 (-18.7563, 23.4956) -> (-16.7432, 19.9912)
  line L551 (-22.7977, 23.5044) -> (-18.7563, 23.4956)
  line L552 (-24.8261, 20.0088) -> (-22.7977, 23.5044)
  line L553 (-22.8129, 16.5044) -> (-24.8261, 20.0088)
  line L554 (-18.7715, 16.4956) -> (-22.8129, 16.5044)
  line L555 (-16.7432, 3.9912) -> (-18.7715, 0.4956)
  line L556 (-18.7563, 7.4956) -> (-16.7432, 3.9912)
  line L557 (-22.7977, 7.5044) -> (-18.7563, 7.4956)
  line L558 (-24.8261, 4.0088) -> (-22.7977, 7.5044)
  line L559 (-22.8129, 0.5044) -> (-24.8261, 4.0088)
  line L560 (-18.7715, 0.4956) -> (-22.8129, 0.5044)
  line L561 (-16.7432, 27.9912) -> (-18.7715, 24.4956)
  line L562 (-18.7563, 31.4956) -> (-16.7432, 27.9912)
  line L563 (-22.7977, 31.5044) -> (-18.7563, 31.4956)
  line L564 (-24.8261, 28.0088) -> (-22.7977, 31.5044)
  line L565 (-22.8129, 24.5044) -> (-24.8261, 28.0088)
  line L566 (-18.7715, 24.4956) -> (-22.8129, 24.5044)
  line L567 (-16.7432, -4.0088) -> (-18.7715, -7.5044)
  line L568 (-18.7563, -0.5044) -> (-16.7432, -4.0088)
  line L569 (-22.7977, -0.4956) -> (-18.7563, -0.5044)
  line L570 (-24.8261, -3.9912) -> (-22.7977, -0.4956)
  line L571 (-22.8129, -7.4956) -> (-24.8261, -3.9912)
  line L572 (-18.7715, -7.5044) -> (-22.8129, -7.4956)
  line L573 (-16.7432, 35.9912) -> (-18.7715, 32.4956)
  line L574 (-18.7563, 39.4956) -> (-16.7432, 35.9912)
  line L575 (-22.7977, 39.5044) -> (-18.7563, 39.4956)
  line L576 (-24.8261, 36.0088) -> (-22.7977, 39.5044)
  line L577 (-22.8129, 32.5044) -> (-24.8261, 36.0088)
  line L578 (-18.7715, 32.4956) -> (-22.8129, 32.5044)
  line L579 (-16.7432, -12.0088) -> (-18.7715, -15.5044)
  line L580 (-18.7563, -8.5044) -> (-16.7432, -12.0088)
  line L581 (-22.7977, -8.4956) -> (-18.7563, -8.5044)
  line L582 (-24.8261, -11.9912) -> (-22.7977, -8.4956)
  line L583 (-22.8129, -15.4956) -> (-24.8261, -11.9912)
  line L584 (-18.7715, -15.5044) -> (-22.8129, -15.4956)
  line L585 (-16.7432, 43.9912) -> (-18.7715, 40.4956)
  line L586 (-18.7563, 47.4956) -> (-16.7432, 43.9912)
  line L587 (-22.7977, 47.5044) -> (-18.7563, 47.4956)
  line L588 (-24.8261, 44.0088) -> (-22.7977, 47.5044)
  line L589 (-22.8129, 40.5044) -> (-24.8261, 44.0088)
  line L590 (-18.7715, 40.4956) -> (-22.8129, 40.5044)
  line L591 (-16.7432, -20.0088) -> (-18.7715, -23.5044)
  line L592 (-18.7563, -16.5044) -> (-16.7432, -20.0088)
  line L593 (-22.7977, -16.4956) -> (-18.7563, -16.5044)
  line L594 (-24.8261, -19.9912) -> (-22.7977, -16.4956)
  line L595 (-22.8129, -23.4956) -> (-24.8261, -19.9912)
  line L596 (-18.7715, -23.5044) -> (-22.8129, -23.4956)
  line L597 (-16.7432, 51.9912) -> (-18.7715, 48.4956)
  line L598 (-18.7563, 55.4956) -> (-16.7432, 51.9912)
  line L599 (-22.7977, 55.5044) -> (-18.7563, 55.4956)
  line L600 (-24.8261, 52.0088) -> (-22.7977, 55.5044)
  line L601 (-22.8129, 48.5044) -> (-24.8261, 52.0088)
  line L602 (-18.7715, 48.4956) -> (-22.8129, 48.5044)
  line L603 (-16.7432, -28.0088) -> (-18.7715, -31.5044)
  line L604 (-18.7563, -24.5044) -> (-16.7432, -28.0088)
  line L605 (-22.7977, -24.4956) -> (-18.7563, -24.5044)
  line L606 (-24.8261, -27.9912) -> (-22.7977, -24.4956)
  line L607 (-22.8129, -31.4956) -> (-24.8261, -27.9912)
  line L608 (-18.7715, -31.5044) -> (-22.8129, -31.4956)
  line L609 (-16.7432, 59.9912) -> (-18.7715, 56.4956)
  line L610 (-18.7563, 63.4956) -> (-16.7432, 59.9912)
  line L611 (-22.7977, 63.5044) -> (-18.7563, 63.4956)
  line L612 (-24.8261, 60.0088) -> (-22.7977, 63.5044)
  line L613 (-22.8129, 56.5044) -> (-24.8261, 60.0088)
  line L614 (-18.7715, 56.4956) -> (-22.8129, 56.5044)
  line L615 (-16.7432, -36.0088) -> (-18.7715, -39.5044)
  line L616 (-18.7563, -32.5044) -> (-16.7432, -36.0088)
  line L617 (-22.7977, -32.4956) -> (-18.7563, -32.5044)
  line L618 (-24.8261, -35.9912) -> (-22.7977, -32.4956)
  line L619 (-22.8129, -39.4956) -> (-24.8261, -35.9912)
  line L620 (-18.7715, -39.5044) -> (-22.8129, -39.4956)
  line L621 (-16.7432, 67.9912) -> (-18.7715, 64.4956)
  line L622 (-18.7563, 71.4956) -> (-16.7432, 67.9912)
  line L623 (-22.7977, 71.5044) -> (-18.7563, 71.4956)
  line L624 (-24.8261, 68.0088) -> (-22.7977, 71.5044)
  line L625 (-22.8129, 64.5044) -> (-24.8261, 68.0088)
  line L626 (-18.7715, 64.4956) -> (-22.8129, 64.5044)
  line L627 (-16.7432, -44.0088) -> (-18.7715, -47.5044)
  line L628 (-18.7563, -40.5044) -> (-16.7432, -44.0088)
  line L629 (-22.7977, -40.4956) -> (-18.7563, -40.5044)
  line L630 (-24.8261, -43.9912) -> (-22.7977, -40.4956)
  line L631 (-22.8129, -47.4956) -> (-24.8261, -43.9912)
  line L632 (-18.7715, -47.5044) -> (-22.8129, -47.4956)
  line L633 (31.7543, -16.0088) -> (29.7259, -19.5044)
  line L634 (29.7411, -12.5044) -> (31.7543, -16.0088)
  line L635 (25.6997, -12.4956) -> (29.7411, -12.5044)
  line L636 (23.6714, -15.9912) -> (25.6997, -12.4956)
  line L637 (25.6845, -19.4956) -> (23.6714, -15.9912)
  line L638 (29.7259, -19.5044) -> (25.6845, -19.4956)
  line L639 (31.7543, -8.0088) -> (29.7259, -11.5044)
  line L640 (29.7411, -4.5044) -> (31.7543, -8.0088)
  line L641 (25.6997, -4.4956) -> (29.7411, -4.5044)
  line L642 (23.6714, -7.9912) -> (25.6997, -4.4956)
  line L643 (25.6845, -11.4956) -> (23.6714, -7.9912)
  line L644 (29.7259, -11.5044) -> (25.6845, -11.4956)
  line L645 (31.7543, -24.0088) -> (29.7259, -27.5044)
  line L646 (29.7411, -20.5044) -> (31.7543, -24.0088)
  line L647 (25.6997, -20.4956) -> (29.7411, -20.5044)
  line L648 (23.6714, -23.9912) -> (25.6997, -20.4956)
  line L649 (25.6845, -27.4956) -> (23.6714, -23.9912)
  line L650 (29.7259, -27.5044) -> (25.6845, -27.4956)
  line L651 (31.7543, -0.0088) -> (29.7259, -3.5044)
  line L652 (29.7411, 3.4956) -> (31.7543, -0.0088)
  line L653 (25.6997, 3.5044) -> (29.7411, 3.4956)
  line L654 (23.6714, 0.0088) -> (25.6997, 3.5044)
  line L655 (25.6845, -3.4956) -> (23.6714, 0.0088)
  line L656 (29.7259, -3.5044) -> (25.6845, -3.4956)
  line L657 (31.7543, -32.0088) -> (29.7259, -35.5044)
  line L658 (29.7411, -28.5044) -> (31.7543, -32.0088)
  line L659 (25.6997, -28.4956) -> (29.7411, -28.5044)
  line L660 (23.6714, -31.9912) -> (25.6997, -28.4956)
  line L661 (25.6845, -35.4956) -> (23.6714, -31.9912)
  line L662 (29.7259, -35.5044) -> (25.6845, -35.4956)
  line L663 (31.7543, 7.9912) -> (29.7259, 4.4956)
  line L664 (29.7411, 11.4956) -> (31.7543, 7.9912)
  line L665 (25.6997, 11.5044) -> (29.7411, 11.4956)
  line L666 (23.6714, 8.0088) -> (25.6997, 11.5044)
  line L667 (25.6845, 4.5044) -> (23.6714, 8.0088)
  line L668 (29.7259, 4.4956) -> (25.6845, 4.5044)
  line L669 (31.7543, -40.0088) -> (29.7259, -43.5044)
  line L670 (29.7411, -36.5044) -> (31.7543, -40.0088)
  line L671 (25.6997, -36.4956) -> (29.7411, -36.5044)
  line L672 (23.6714, -39.9912) -> (25.6997, -36.4956)
  line L673 (25.6845, -43.4956) -> (23.6714, -39.9912)
  line L674 (29.7259, -43.5044) -> (25.6845, -43.4956)
  line L675 (31.7543, 15.9912) -> (29.7259, 12.4956)
  line L676 (29.7411, 19.4956) -> (31.7543, 15.9912)
  line L677 (25.6997, 19.5044) -> (29.7411, 19.4956)
  line L678 (23.6714, 16.0088) -> (25.6997, 19.5044)
  line L679 (25.6845, 12.5044) -> (23.6714, 16.0088)
  line L680 (29.7259, 12.4956) -> (25.6845, 12.5044)
  line L681 (31.7543, -48.0088) -> (29.7259, -51.5044)
  line L682 (29.7411, -44.5044) -> (31.7543, -48.0088)
  line L683 (25.6997, -44.4956) -> (29.7411, -44.5044)
  line L684 (23.6714, -47.9912) -> (25.6997, -44.4956)
  line L685 (25.6845, -51.4956) -> (23.6714, -47.9912)
  line L686 (29.7259, -51.5044) -> (25.6845, -51.4956)
  line L687 (31.7543, 23.9912) -> (29.7259, 20.4956)
  line L688 (29.7411, 27.4956) -> (31.7543, 23.9912)
  line L689 (25.6997, 27.5044) -> (29.7411, 27.4956)
  line L690 (23.6714, 24.0088) -> (25.6997, 27.5044)
  line L691 (25.6845, 20.5044) -> (23.6714, 24.0088)
  line L692 (29.7259, 20.4956) -> (25.6845, 20.5044)
  line L693 (31.7543, -56.0088) -> (29.7259, -59.5044)
  line L694 (29.7411, -52.5044) -> (31.7543, -56.0088)
  line L695 (25.6997, -52.4956) -> (29.7411, -52.5044)
  line L696 (23.6714, -55.9912) -> (25.6997, -52.4956)
  line L697 (25.6845, -59.4956) -> (23.6714, -55.9912)
  line L698 (29.7259, -59.5044) -> (25.6845, -59.4956)
  line L699 (31.7543, 31.9912) -> (29.7259, 28.4956)
  line L700 (29.7411, 35.4956) -> (31.7543, 31.9912)
  line L701 (25.6997, 35.5044) -> (29.7411, 35.4956)
  line L702 (23.6714, 32.0088) -> (25.6997, 35.5044)
  line L703 (25.6845, 28.5044) -> (23.6714, 32.0088)
  line L704 (29.7259, 28.4956) -> (25.6845, 28.5044)
  line L705 (31.7543, -64.0088) -> (29.7259, -67.5044)
  line L706 (29.7411, -60.5044) -> (31.7543, -64.0088)
  line L707 (25.6997, -60.4956) -> (29.7411, -60.5044)
  line L708 (23.6714, -63.9912) -> (25.6997, -60.4956)
  line L709 (25.6845, -67.4956) -> (23.6714, -63.9912)
  line L710 (29.7259, -67.5044) -> (25.6845, -67.4956)
  line L711 (31.7543, 39.9912) -> (29.7259, 36.4956)
  line L712 (29.7411, 43.4956) -> (31.7543, 39.9912)
  line L713 (25.6997, 43.5044) -> (29.7411, 43.4956)
  line L714 (23.6714, 40.0088) -> (25.6997, 43.5044)
  line L715 (25.6845, 36.5044) -> (23.6714, 40.0088)
  line L716 (29.7259, 36.4956) -> (25.6845, 36.5044)
  line L717 (31.7543, -72.0088) -> (29.7259, -75.5044)
  line L718 (29.7411, -68.5044) -> (31.7543, -72.0088)
  line L719 (25.6997, -68.4956) -> (29.7411, -68.5044)
  line L720 (23.6714, -71.9912) -> (25.6997, -68.4956)
  line L721 (25.6845, -75.4956) -> (23.6714, -71.9912)
  line L722 (29.7259, -75.5044) -> (25.6845, -75.4956)
  line L723 (-23.6714, 15.9912) -> (-25.6997, 12.4956)
  line L724 (-25.6845, 19.4956) -> (-23.6714, 15.9912)
  line L725 (-29.7259, 19.5044) -> (-25.6845, 19.4956)
  line L726 (-31.7543, 16.0088) -> (-29.7259, 19.5044)
  line L727 (-29.7411, 12.5044) -> (-31.7543, 16.0088)
  line L728 (-25.6997, 12.4956) -> (-29.7411, 12.5044)
  line L729 (-23.6714, 23.9912) -> (-25.6997, 20.4956)
  line L730 (-25.6845, 27.4956) -> (-23.6714, 23.9912)
  line L731 (-29.7259, 27.5044) -> (-25.6845, 27.4956)
  line L732 (-31.7543, 24.0088) -> (-29.7259, 27.5044)
  line L733 (-29.7411, 20.5044) -> (-31.7543, 24.0088)
  line L734 (-25.6997, 20.4956) -> (-29.7411, 20.5044)
  line L735 (-23.6714, 7.9912) -> (-25.6997, 4.4956)
  line L736 (-25.6845, 11.4956) -> (-23.6714, 7.9912)
  line L737 (-29.7259, 11.5044) -> (-25.6845, 11.4956)
  line L738 (-31.7543, 8.0088) -> (-29.7259, 11.5044)
  line L739 (-29.7411, 4.5044) -> (-31.7543, 8.0088)
  line L740 (-25.6997, 4.4956) -> (-29.7411, 4.5044)
  line L741 (-23.6714, 31.9912) -> (-25.6997, 28.4956)
  line L742 (-25.6845, 35.4956) -> (-23.6714, 31.9912)
  line L743 (-29.7259, 35.5044) -> (-25.6845, 35.4956)
  line L744 (-31.7543, 32.0088) -> (-29.7259, 35.5044)
  line L745 (-29.7411, 28.5044) -> (-31.7543, 32.0088)
  line L746 (-25.6997, 28.4956) -> (-29.7411, 28.5044)
  line L747 (-23.6714, -0.0088) -> (-25.6997, -3.5044)
  line L748 (-25.6845, 3.4956) -> (-23.6714, -0.0088)
  line L749 (-29.7259, 3.5044) -> (-25.6845, 3.4956)
  line L750 (-31.7543, 0.0088) -> (-29.7259, 3.5044)
  line L751 (-29.7411, -3.4956) -> (-31.7543, 0.0088)
  line L752 (-25.6997, -3.5044) -> (-29.7411, -3.4956)
  line L753 (-23.6714, 39.9912) -> (-25.6997, 36.4956)
  line L754 (-25.6845, 43.4956) -> (-23.6714, 39.9912)
  line L755 (-29.7259, 43.5044) -> (-25.6845, 43.4956)
  line L756 (-31.7543, 40.0088) -> (-29.7259, 43.5044)
  line L757 (-29.7411, 36.5044) -> (-31.7543, 40.0088)
  line L758 (-25.6997, 36.4956) -> (-29.7411, 36.5044)
  line L759 (-23.6714, -8.0088) -> (-25.6997, -11.5044)
  line L760 (-25.6845, -4.5044) -> (-23.6714, -8.0088)
  line L761 (-29.7259, -4.4956) -> (-25.6845, -4.5044)
  line L762 (-31.7543, -7.9912) -> (-29.7259, -4.4956)
  line L763 (-29.7411, -11.4956) -> (-31.7543, -7.9912)
  line L764 (-25.6997, -11.5044) -> (-29.7411, -11.4956)
  line L765 (-23.6714, 47.9912) -> (-25.6997, 44.4956)
  line L766 (-25.6845, 51.4956) -> (-23.6714, 47.9912)
  line L767 (-29.7259, 51.5044) -> (-25.6845, 51.4956)
  line L768 (-31.7543, 48.0088) -> (-29.7259, 51.5044)
  line L769 (-29.7411, 44.5044) -> (-31.7543, 48.0088)
  line L770 (-25.6997, 44.4956) -> (-29.7411, 44.5044)
  line L771 (-23.6714, -16.0088) -> (-25.6997, -19.5044)
  line L772 (-25.6845, -12.5044) -> (-23.6714, -16.0088)
  line L773 (-29.7259, -12.4956) -> (-25.6845, -12.5044)
  line L774 (-31.7543, -15.9912) -> (-29.7259, -12.4956)
  line L775 (-29.7411, -19.4956) -> (-31.7543, -15.9912)
  line L776 (-25.6997, -19.5044) -> (-29.7411, -19.4956)
  line L777 (-23.6714, 55.9912) -> (-25.6997, 52.4956)
  line L778 (-25.6845, 59.4956) -> (-23.6714, 55.9912)
  line L779 (-29.7259, 59.5044) -> (-25.6845, 59.4956)
  line L780 (-31.7543, 56.0088) -> (-29.7259, 59.5044)
  line L781 (-29.7411, 52.5044) -> (-31.7543, 56.0088)
  line L782 (-25.6997, 52.4956) -> (-29.7411, 52.5044)
  line L783 (-23.6714, -24.0088) -> (-25.6997, -27.5044)
  line L784 (-25.6845, -20.5044) -> (-23.6714, -24.0088)
  line L785 (-29.7259, -20.4956) -> (-25.6845, -20.5044)
  line L786 (-31.7543, -23.9912) -> (-29.7259, -20.4956)
  line L787 (-29.7411, -27.4956) -> (-31.7543, -23.9912)
  line L788 (-25.6997, -27.5044) -> (-29.7411, -27.4956)
  line L789 (-23.6714, 63.9912) -> (-25.6997, 60.4956)
  line L790 (-25.6845, 67.4956) -> (-23.6714, 63.9912)
  line L791 (-29.7259, 67.5044) -> (-25.6845, 67.4956)
  line L792 (-31.7543, 64.0088) -> (-29.7259, 67.5044)
  line L793 (-29.7411, 60.5044) -> (-31.7543, 64.0088)
  line L794 (-25.6997, 60.4956) -> (-29.7411, 60.5044)
  line L795 (-23.6714, -32.0088) -> (-25.6997, -35.5044)
  line L796 (-25.6845, -28.5044) -> (-23.6714, -32.0088)
  line L797 (-29.7259, -28.4956) -> (-25.6845, -28.5044)
  line L798 (-31.7543, -31.9912) -> (-29.7259, -28.4956)
  line L799 (-29.7411, -35.4956) -> (-31.7543, -31.9912)
  line L800 (-25.6997, -35.5044) -> (-29.7411, -35.4956)
  line L801 (-23.6714, 71.9912) -> (-25.6997, 68.4956)
  line L802 (-25.6845, 75.4956) -> (-23.6714, 71.9912)
  line L803 (-29.7259, 75.5044) -> (-25.6845, 75.4956)
  line L804 (-31.7543, 72.0088) -> (-29.7259, 75.5044)
  line L805 (-29.7411, 68.5044) -> (-31.7543, 72.0088)
  line L806 (-25.6997, 68.4956) -> (-29.7411, 68.5044)
  line L807 (-23.6714, -40.0088) -> (-25.6997, -43.5044)
  line L808 (-25.6845, -36.5044) -> (-23.6714, -40.0088)
  line L809 (-29.7259, -36.4956) -> (-25.6845, -36.5044)
  line L810 (-31.7543, -39.9912) -> (-29.7259, -36.4956)
  line L811 (-29.7411, -43.4956) -> (-31.7543, -39.9912)
  line L812 (-25.6997, -43.5044) -> (-29.7411, -43.4956)
  line L813 (38.6825, -20.0088) -> (36.6541, -23.5044)
  line L814 (36.6693, -16.5044) -> (38.6825, -20.0088)
  line L815 (32.6279, -16.4956) -> (36.6693, -16.5044)
  line L816 (30.5996, -19.9912) -> (32.6279, -16.4956)
  line L817 (32.6127, -23.4956) -> (30.5996, -19.9912)
  line L818 (36.6541, -23.5044) -> (32.6127, -23.4956)
  line L819 (38.6825, -12.0088) -> (36.6541, -15.5044)
  line L820 (36.6693, -8.5044) -> (38.6825, -12.0088)
  line L821 (32.6279, -8.4956) -> (36.6693, -8.5044)
  line L822 (30.5996, -11.9912) -> (32.6279, -8.4956)
  line L823 (32.6127, -15.4956) -> (30.5996, -11.9912)
  line L824 (36.6541, -15.5044) -> (32.6127, -15.4956)
  line L825 (38.6825, -28.0088) -> (36.6541, -31.5044)
  line L826 (36.6693, -24.5044) -> (38.6825, -28.0088)
  line L827 (32.6279, -24.4956) -> (36.6693, -24.5044)
  line L828 (30.5996, -27.9912) -> (32.6279, -24.4956)
  line L829 (32.6127, -31.4956) -> (30.5996, -27.9912)
  line L830 (36.6541, -31.5044) -> (32.6127, -31.4956)
  line L831 (38.6825, -4.0088) -> (36.6541, -7.5044)
  line L832 (36.6693, -0.5044) -> (38.6825, -4.0088)
  line L833 (32.6279, -0.4956) -> (36.6693, -0.5044)
  line L834 (30.5996, -3.9912) -> (32.6279, -0.4956)
  line L835 (32.6127, -7.4956) -> (30.5996, -3.9912)
  line L836 (36.6541, -7.5044) -> (32.6127, -7.4956)
  line L837 (38.6825, -36.0088) -> (36.6541, -39.5044)
  line L838 (36.6693, -32.5044) -> (38.6825, -36.0088)
  line L839 (32.6279, -32.4956) -> (36.6693, -32.5044)
  line L840 (30.5996, -35.9912) -> (32.6279, -32.4956)
  line L841 (32.6127, -39.4956) -> (30.5996, -35.9912)
  line L842 (36.6541, -39.5044) -> (32.6127, -39.4956)
  line L843 (38.6825, 3.9912) -> (36.6541, 0.4956)
  line L844 (36.6693, 7.4956) -> (38.6825, 3.9912)
  line L845 (32.6279, 7.5044) -> (36.6693, 7.4956)
  line L846 (30.5996, 4.0088) -> (32.6279, 7.5044)
  line L847 (32.6127, 0.5044) -> (30.5996, 4.0088)
  line L848 (36.6541, 0.4956) -> (32.6127, 0.5044)
  line L849 (38.6825, -44.0088) -> (36.6541, -47.5044)
  line L850 (36.6693, -40.5044) -> (38.6825, -44.0088)
  line L851 (32.6279, -40.4956) -> (36.6693, -40.5044)
  line L852 (30.5996, -43.9912) -> (32.6279, -40.4956)
  line L853 (32.6127, -47.4956) -> (30.5996, -43.9912)
  line L854 (36.6541, -47.5044) -> (32.6127, -47.4956)
  line L855 (38.6825, 11.9912) -> (36.6541, 8.4956)
  line L856 (36.6693, 15.4956) -> (38.6825, 11.9912)
  line L857 (32.6279, 15.5044) -> (36.6693, 15.4956)
  line L858 (30.5996, 12.0088) -> (32.6279, 15.5044)
  line L859 (32.6127, 8.5044) -> (30.5996, 12.0088)
  line L860 (36.6541, 8.4956) -> (32.6127, 8.5044)
  line L861 (38.6825, -52.0088) -> (36.6541, -55.5044)
  line L862 (36.6693, -48.5044) -> (38.6825, -52.0088)
  line L863 (32.6279, -48.4956) -> (36.6693, -48.5044)
  line L864 (30.5996, -51.9912) -> (32.6279, -48.4956)
  line L865 (32.6127, -55.4956) -> (30.5996, -51.9912)
  line L866 (36.6541, -55.5044) -> (32.6127, -55.4956)
  line L867 (38.6825, 19.9912) -> (36.6541, 16.4956)
  line L868 (36.6693, 23.4956) -> (38.6825, 19.9912)
  line L869 (32.6279, 23.5044) -> (36.6693, 23.4956)
  line L870 (30.5996, 20.0088) -> (32.6279, 23.5044)
  line L871 (32.6127, 16.5044) -> (30.5996, 20.0088)
  line L872 (36.6541, 16.4956) -> (32.6127, 16.5044)
  line L873 (38.6825, -60.0088) -> (36.6541, -63.5044)
  line L874 (36.6693, -56.5044) -> (38.6825, -60.0088)
  line L875 (32.6279, -56.4956) -> (36.6693, -56.5044)
  line L876 (30.5996, -59.9912) -> (32.6279, -56.4956)
  line L877 (32.6127, -63.4956) -> (30.5996, -59.9912)
  line L878 (36.6541, -63.5044) -> (32.6127, -63.4956)
  line L879 (38.6825, 27.9912) -> (36.6541, 24.4956)
  line L880 (36.6693, 31.4956) -> (38.6825, 27.9912)
  line L881 (32.6279, 31.5044) -> (36.6693, 31.4956)
  line L882 (30.5996, 28.0088) -> (32.6279, 31.5044)
  line L883 (32.6127, 24.5044) -> (30.5996, 28.0088)
  line L884 (36.6541, 24.4956) -> (32.6127, 24.5044)
  line L885 (38.6825, -68.0088) -> (36.6541, -71.5044)
  line L886 (36.6693, -64.5044) -> (38.6825, -68.0088)
  line L887 (32.6279, -64.4956) -> (36.6693, -64.5044)
  line L888 (30.5996, -67.9912) -> (32.6279, -64.4956)
  line L889 (32.6127, -71.4956) -> (30.5996, -67.9912)
  line L890 (36.6541, -71.5044) -> (32.6127, -71.4956)
  line L891 (38.6825, 35.9912) -> (36.6541, 32.4956)
  line L892 (36.6693, 39.4956) -> (38.6825, 35.9912)
  line L893 (32.6279, 39.5044) -> (36.6693, 39.4956)
  line L894 (30.5996, 36.0088) -> (32.6279, 39.5044)
  line L895 (32.6127, 32.5044) -> (30.5996, 36.0088)
  line L896 (36.6541, 32.4956) -> (32.6127, 32.5044)
  line L897 (38.6825, -76.0088) -> (36.6541, -79.5044)
  line L898 (36.6693, -72.5044) -> (38.6825, -76.0088)
  line L899 (32.6279, -72.4956) -> (36.6693, -72.5044)
  line L900 (30.5996, -75.9912) -> (32.6279, -72.4956)